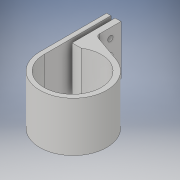
# Autodesk Inventor part: MotorMountB
Saved by Autodesk Inventor 2018 (Build 220112000, 112)
## iProperties
Created: 2018-01-25
Part Number: MotorMountB
Material: Generic
Document SubType Name: Modeling
Designer: Mira
Density: 1 g/cm^3
Appearance: Default
Author: Mira
Autodesk Inventor part; units mm, degrees
ref_plane "YZ Plane" through (0, 0, 0) normal (1, 0, 0) x (0, 1, 0)
ref_plane "XZ Plane" through (0, 0, 0) normal (0, 1, 0) x (-1, 0, 0)
ref_plane "XY Plane" through (0, 0, 0) normal (0, 0, 1) x (1, 0, 0)
sketch "Sketch7" plane through (0, 0, 0) normal (0, 1, 0) x (-1, 0, 0)
  arc A0 (19.304, 0.0015) -> (-6.0429, -17.7596) centre (0.2553, 0.2192) ccw
  line L0 (22.225, -44.45) -> (22.225, 0)
  arc A1 (22.225, 0) -> (-7.3478, -20.9752) centre (0, 0) ccw
  line L1 (-7.3478, -20.9752) -> (10.5747, -27.2537)
  arc A2 (12.7, -30.2501) -> (10.5747, -27.2537) centre (9.525, -30.2501) ccw
  line L2 (12.7, -30.2501) -> (12.7, -44.45)
  line L3 (16.617, -44.45) -> (16.617, -25.6976)
  line L4 (19.304, -22.225) -> (19.304, -44.45)
  line L5 (16.617, -25.6976) -> (16.8723, -25.787)
  line L6 (19.304, -22.225) -> (19.304, 0.0015)
  line L7 (12.7, -44.45) -> (16.617, -44.45)
  line L8 (19.304, -44.45) -> (22.225, -44.45)
  arc A3 (19.304, 0.0015) -> (10.5747, -15.7937) centre (0.2553, 0.2192) ccw
  line L9 (16.617, -25.6976) -> (16.617, -15.7937)
  line L10 (10.5747, -15.7937) -> (16.617, -15.7937)
  point P0 (0, 0)
  point P1 (0, 0)
  constraints: 22 end point, 8 point on circle, 4 centre point, 2 parallel, 1 coincident, 1 collinear, 1 concentric, 1 perpendicular, 1 tangent, 1 vertical
extrude "Extrusion8" add sketch "Sketch7" along normal blind 33.02
sketch "Sketch8" plane through (-12.7, 0, -30.2501) normal (1, 0, 0) x (0, 0, -1)
  circle A0 centre (7.0999, 26.67) radius 1.8034
  line L0 (0, 0) -> (0, 25.4) construction
  line L1 (0, 24.4432) -> (14.1999, 24.4432) construction
  line L2 (14.1999, 24.4432) -> (7.0999, 24.4432) construction
  line L3 (7.0999, 24.4432) -> (7.0999, 0) construction
  line L4 (14.1999, 0) -> (-30.2501, 0) construction
  circle A1 centre (7.0999, 16.51) radius 1.8034
  circle A2 centre (7.0999, 6.35) radius 1.8034
  line L5 (14.1999, 0) -> (14.1999, 33.02)
  line L6 (14.1999, 16.51) -> (0, 16.51) construction
  dimension "d35" = 3.6068
  dimension "d36" = 3.6068
  dimension "d37" = 3.6068
  dimension "d38" = 10.16
  dimension "d39" = 10.16
  constraints: 14 end point, 6 point on line, 3 centre point, 3 midpoint, 2 perpendicular, 1 horizontal
  measures "d35" diameter of A0
  measures "d36" diameter of A1
  measures "d37" diameter of A2
  measures "d38" distance of A0.centre A1.centre
  measures "d39" distance of A2.centre A1.centre
extrude "Extrusion9" cut sketch "Sketch8" against normal through all
body "Solid2"
